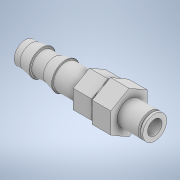
# Autodesk Inventor part: sambungan cilek ng gede
Saved by Autodesk Inventor 2021 (Build 250183000, 183)
## iProperties
Created: 2023-10-16
Part Number: sambungan cilek ng gede
Material: Generic
Document SubType Name: Modeling
Designer: user
Density: 1 g/cm^3
Appearance: Default
Author: user
Autodesk Inventor part; units mm, degrees
ref_plane "YZ Plane" through (0, 0, 0) normal (1, 0, 0) x (0, 1, 0)
ref_plane "XZ Plane" through (0, 0, 0) normal (0, 1, 0) x (-1, 0, 0)
ref_plane "XY Plane" through (0, 0, 0) normal (0, 0, 1) x (1, 0, 0)
sketch "Sketch1" plane through (0, 0, 0) normal (0, 0, 1) x (1, 0, 0)
  line L0 (-20, 4.75) -> (-20, 5.7007)
  line L1 (-20, 5.7007) -> (-25, 4.75)
  line L2 (-20, 4.75) -> (-15, 4.75)
  line L3 (-10, 6.0299) -> (-15, 4.75)
  line L4 (-10, 5.3899) -> (0, 5.3899)
  line L5 (-10, 6.0299) -> (-10, 5.3899)
  line L6 (-27.5, 4.75) -> (-27.5, 4)
  line L7 (-27.5, 4.75) -> (-25, 4.75)
  line L8 (-27.5, 4) -> (0, 4)
  line L9 (0, 8) -> (8, 8)
  line L10 (0, 8) -> (0, 5.3899)
  line L11 (8, 8) -> (8, 7)
  line L12 (8, 7) -> (9, 7)
  line L13 (9, 9) -> (17, 9)
  line L14 (26, 3.1165) -> (0, 3.1165)
  line L15 (0, 4) -> (0, 3.1165)
  line L16 (9, 9) -> (9, 7)
  line L17 (26, 4) -> (26, 5.1165)
  line L18 (26, 5.1165) -> (17, 5.1165)
  line L19 (17, 5.1165) -> (17, 9)
  line L20 (26, 4) -> (27, 4)
  line L21 (27, 4) -> (27, 5.1165)
  line L22 (27, 5.1165) -> (28, 5.1165)
  line L23 (28, 5.1165) -> (28, 3.1165)
  line L24 (28, 3.1165) -> (26, 3.1165)
  line L25 (-35.0249, 0) -> (33.4829, 0)
  point P0 (0, 0)
  point P1 (0, 4.75)
  point P2 (13, 7)
  dimension "d3" = 5
  dimension "d4" = 5
  dimension "d14" = 0.75
  dimension "d15" = 1
  dimension "d16" = 8
  dimension "d26" = 2
  dimension "d27" = 1
  dimension "d28" = 1
  constraints: 52 end point, 7 horizontal, 6 perpendicular, 5 vertical, 1 parallel
  measures "d3" distance of L1.end L0.start
  measures "d4" distance of L0.start L2.end
  measures "d14" distance between parallel lines of L8 L7
  measures "d15" distance of L11.end L12.end
  measures "d16" distance of L13.start L13.end
  measures "d26" distance of L14.start L17.end
  measures "d27" distance of L17.start L20.end
  measures "d28" distance of L21.end L22.end
sketch "Sketch2" plane through (0, 0, 0) normal (0, 0, 1) x (1, 0, 0)
  point P0 (0, 0)
sketch "Sketch3" plane through (0, 0, 0) normal (0, 0, 1) x (1, 0, 0)
  point P0 (0, 0)
sketch "Sketch4" plane through (0, 0, 0) normal (0, 0, 1) x (1, 0, 0)
  point P0 (0, 0)
sketch "Sketch5" plane through (0, 0, 0) normal (1, 0, 0) x (0, 1, 0)
  point P0 (0, 0)
sketch "Sketch6" plane through (0, 0, 0) normal (0, 0, 1) x (1, 0, 0)
  line L0 (8.9873, 9.0104) -> (8.9873, 6.9688)
  point P0 (0, 0)
  constraints: 2 end point, 1 vertical
sketch "Sketch7" plane through (0, 0, 0) normal (0, 0, 1) x (1, 0, 0)
  point P0 (0, 0)
sketch "Sketch8" plane through (0, 0, 0) normal (0, 0, 1) x (1, 0, 0)
  point P0 (0, 0)
revolve "Revolution1" add sketch "Sketch1" angle 360 about axis through (-35.0249, 0, 0) along (1, 0, 0)
sketch "Sketch9" plane through (17, 0, 0) normal (1, 0, 0) x (0, 0, -1)
  circle A0 centre (0, 0) radius 7 projected
  circle A1 centre (0, 0) radius 9 projected
  circle A2 centre (0, 0) radius 9 projected
  circle A3 centre (0, 0) radius 5.1165 projected
  circle A4 centre (0, 0) radius 3.1165 projected
  circle A5 centre (0, 0) radius 5.7007 projected
  line L0 (0, 9) -> (7.7942, 4.5)
  line L1 (7.7942, 4.5) -> (7.7942, -4.5)
  line L2 (7.7942, -4.5) -> (0, -9)
  line L3 (0, -9) -> (-7.7942, -4.5)
  line L4 (-7.7942, -4.5) -> (-7.7942, 4.5)
  line L5 (-7.7942, 4.5) -> (0, 9)
  point P0 (0, -9)
  point P1 (0, -9)
  point P2 (7.7942, -4.5)
  point P3 (7.7942, -4.5)
  constraints: 12 end point, 1 coincident, 1 vertical alignment, 14 other
extrude "Extrusion1" cut sketch "Sketch9" against normal blind 8 contours A1 L1 | L0 A1 | A1 L2 | L5 A1 | A1 L3 | L4 A1
sketch "Sketch10" plane through (0, 0, 0) normal (-1, 0, 0) x (0, 0, 1)
  circle A0 centre (0, 0) radius 5.3899 projected
  circle A1 centre (0, 0) radius 8 projected
  circle A2 centre (0, 0) radius 3.1165 projected
  circle A3 centre (0, 0) radius 4 projected
  circle A4 centre (0, 0) radius 5.3899 projected
  circle A5 centre (0, 0) radius 8 projected
  circle A6 centre (0, 0) radius 3.1165 projected
  circle A7 centre (0, 0) radius 4 projected
  circle A8 centre (0, 0) radius 8 projected
  line L0 (6.9282, -4) -> (0, -8)
  line L1 (0, -8) -> (-6.9282, -4)
  line L2 (-6.9282, -4) -> (-6.9282, 4)
  line L3 (-6.9282, 4) -> (0, 8)
  line L4 (0, 8) -> (6.9282, 4)
  line L5 (6.9282, 4) -> (6.9282, -4)
  point P0 (0, 8)
  point P1 (0, 8)
  point P2 (-6.9282, 4)
  point P3 (-6.9282, 4)
  point P4 (0, -8)
  point P5 (0, -8)
  constraints: 12 end point, 1 coincident, 15 other
extrude "Extrusion2" cut sketch "Sketch10" against normal blind 8 contours A1 L5 | L4 A1 | A1 L0 | L3 A1 | A1 L1 | L2 A1
chamfer "Chamfer1" distance 0.2 angle 45 1 edges at (-20, -5.7007, 0)
chamfer "Chamfer2" distance 0.2 angle 45 1 edges at (-10, -6.0299, 0)
body "Solid1"
